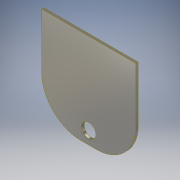
# Autodesk Inventor part: clamp
Saved by Autodesk Inventor 2019 (Build 230136000, 136)
## iProperties
Created: 2020-02-11
Part Number: clamp
Material: Generic
Document SubType Name: Modeling
Designer: Vinayak
Density: 1 g/cm^3
Appearance: Silver
Author: Vinayak
Autodesk Inventor part; units mm, degrees
ref_plane "YZ Plane" through (0, 0, 0) normal (1, 0, 0) x (0, 1, 0)
ref_plane "XZ Plane" through (0, 0, 0) normal (0, 1, 0) x (-1, 0, 0)
ref_plane "XY Plane" through (0, 0, 0) normal (0, 0, 1) x (1, 0, 0)
sketch "Sketch1" plane through (0, 0, 0) normal (0, 0, 1) x (1, 0, 0)
  line L0 (-25, 0) -> (-35, 0)
  line L1 (-60, 25) -> (-60, 60)
  line L2 (-60, 60) -> (0, 60)
  line L3 (0, 60) -> (0, 25)
  arc A0 (-25, 0) -> (0, 25) centre (-25, 25) ccw
  arc A1 (-60, 25) -> (-35, 0) centre (-35, 25) ccw
  point P0 (0, 0)
  point P1 (-60, 0)
  dimension "d0" = 60
  dimension "d1" = 60
  dimension "d9" = 25
  constraints: 8 end point, 4 point on circle, 4 point on line, 4 tangent, 2 centre point, 2 parallel, 1 equal radius, 1 horizontal, 1 perpendicular
  measures "d0" distance of L1.end L2.end
  measures "d1" distance of point (-60, 0) L1.end
  measures "d9" radius of A0
extrude "Extrusion1" add sketch "Sketch1" along normal blind 1.5
sketch "Sketch2" plane through (0, 0, 1.5) normal (0, 0, 1) x (1, 0, 0)
  line L0 (0, 0) -> (-30, 0)
  line L1 (-35, 0) -> (0, 0) projected
  line L2 (-30, 3.5) -> (-30, 8)
  circle A0 centre (-30, 8) radius 4.5
  point P0 (-60, 0)
  dimension "d6" = 9
  dimension "d4" = 30
  dimension "d5" = 8
  constraints: 4 end point, 1 coincident, 1 point on line, 1 vertical, 1 vertical alignment, 2 other
  measures "d4" distance of L0.start L0.end
  measures "d5" distance of L0.end L2.end
extrude "Extrusion2" cut sketch "Sketch2" against normal blind 1.5
body "Solid1"
